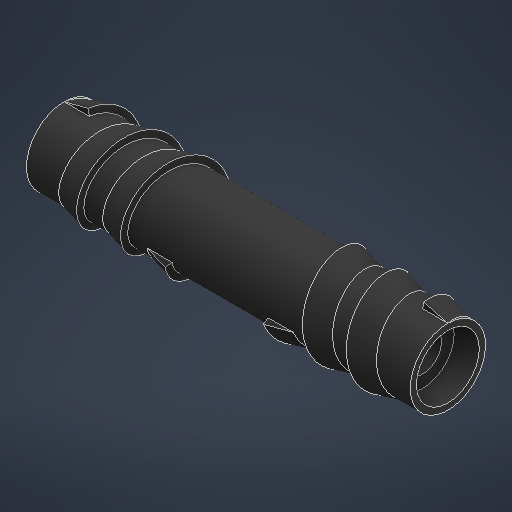
# Autodesk Inventor part: Dribblerschnecke
Saved by Autodesk Inventor 2025.2 (Build 292293000, 293)
## iProperties
Created: 2025-02-12
Part Number: Dribblerschnecke
Material: Generisch
Document SubType Name: Modeling
Designer: Faabs
Density: 1 g/cm^3
Appearance: Gummi - Schwarz
Author: Faabs
Autodesk Inventor part; units mm, degrees
ref_plane "YZ Plane" through (0, 0, 0) normal (1, 0, 0) x (0, 1, 0)
ref_plane "XZ Plane" through (0, 0, 0) normal (0, 1, 0) x (-1, 0, 0)
ref_plane "XY Plane" through (0, 0, 0) normal (0, 0, 1) x (1, 0, 0)
sketch "Skizze1" plane through (0, 0, 0) normal (1, 0, 0) x (0, 1, 0)
  circle A0 centre (0, 0) radius 6
  circle A1 centre (0, 0) radius 3
  dimension "d0" = 12
  dimension "d1" = 6
  constraints: 2 centre point, 2 coincident
  measures "d0" diameter of A0
  measures "d1" diameter of A1
extrude "Extrusion1" add sketch "Skizze1" along normal blind 30.55
sketch "Skizze2" plane through (0, 0, 0) normal (0, 1, 0) x (-1, 0, 0)
  line L0 (-30.55, 6) -> (-30.55, -6) construction
  line L1 (-30.55, 6) -> (-30.55, -6) construction
  line L2 (-30.55, 6) -> (-26.55, 6)
  line L3 (0, 6) -> (-30.55, 6) projected
  line L4 (-30.55, 6) -> (-30.55, 6.1)
  line L5 (-30.55, 6) -> (-26.7263, 7)
  line L6 (-26.7263, 7) -> (-26.55, 6)
  point P0 (0, 0)
  dimension "d4" = 4
  dimension "d5" = 0.1
  dimension "d6" = 80
  dimension "d7" = 1
  constraints: 10 end point, 2 vertical, 1 point on line
  measures "d4" distance of L0.start L2.end
  measures "d5" distance of L3.end L4.end
  measures "d6" angle of L2 L6
  measures "d7" distance from line of L2 L5.end
coil "Spirale1" sketch "Skizze2" operation add axis through (-10, 0, 0) along (-1, 0, 0) pitch 7 turns 2.7 hand right
mirror "Spiegeln1" about plane through (0, 0, 0) normal (1, 0, 0) of "Extrusion1", "Spirale1"
sketch "Skizze3" plane through (30.55, 0, 0) normal (1, 0, 0) x (0, 0, -1)
  circle A0 centre (0, 0) radius 5
  dimension "d16" = 10
  constraints: 1 centre point, 1 coincident
  measures "d16" diameter of A0
extrude "Extrusion2" cut sketch "Skizze3" against normal blind 4
